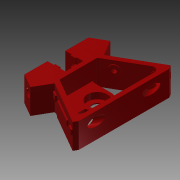
# Autodesk Inventor part: top corner
Saved by Autodesk Inventor 2015 SP1 (Build 190203100, 203)
## iProperties
Created: 2015-01-28
Part Number: top corner
Material: Generic
Document SubType Name: Modeling
Designer: Joseph
Density: 1 g/cm^3
Appearance: Red
Author: Joseph
Autodesk Inventor part; units mm, degrees
note: some values were not read from the file. Chosen so that the rebuilt part matches the saved one: direction of "Hole8".
sketch "Sketch1" plane through (0, 0, 0) normal (0, 0, 1) x (1, 0, 0)
  line L0 (7.9588, 40.9294) -> (17.9588, 23.6089)
  line L1 (17.9588, 23.6089) -> (65.5902, 51.1089)
  line L2 (7.9588, -48.8207) -> (17.9588, -31.5002)
  line L3 (17.9588, -31.5002) -> (65.5902, -59.0002)
  line L4 (65.5902, -59.0002) -> (68.0902, -54.6701)
  line L5 (65.5902, 51.1089) -> (68.0902, 46.7788)
  line L6 (17.039, 17.3044) -> (17.039, -25.1956)
  line L7 (-7.6578, 31.9131) -> (7.9588, 40.9294)
  line L8 (7.9588, -48.8207) -> (-7.6578, -39.8044)
  line L9 (63.0902, 43.892) -> (63.0902, -51.7833)
  line L10 (68.0902, 46.7788) -> (68.0902, -54.6701)
  line L11 (63.0902, 43.892) -> (17.039, 17.3044)
  line L12 (63.0902, -51.7833) -> (17.039, -25.1956)
  line L13 (63.0902, -12.2336) -> (68.0902, -12.2336) construction
  line L14 (63.0902, -51.7833) -> (60.5902, -56.1134) construction
  line L15 (63.0902, 43.892) -> (60.5902, 48.2222) construction
  line L16 (17.039, -3.9456) -> (63.0902, -3.9456) construction
  line L17 (-7.6578, 6.0639) -> (-7.6578, -13.9552) construction
  line L18 (-7.6578, 31.9131) -> (-7.6578, 6.0639)
  line L19 (-7.6578, -13.9552) -> (-7.6578, -39.8044)
  line L20 (-7.6578, -13.9552) -> (-0.4078, -13.9552)
  line L21 (5.0922, -13.9361) -> (12.3422, -13.9361)
  line L22 (12.3422, 6.0639) -> (5.0922, 6.0639)
  line L23 (-0.4078, 6.0639) -> (-7.6578, 6.0639)
  line L24 (12.3422, -6.6861) -> (10.8613, -6.6861)
  line L25 (10.8613, -6.6861) -> (10.8613, -1.1861)
  line L26 (10.8613, -1.1861) -> (12.3422, -1.1861)
  line L27 (5.0922, 6.0639) -> (5.0922, 4.5831)
  line L28 (5.0922, 4.5831) -> (-0.4078, 4.5831)
  line L29 (-0.4078, 4.5831) -> (-0.4078, 6.0639)
  line L30 (-0.4078, -13.9552) -> (-0.4078, -12.4552)
  line L31 (-0.4078, -12.4552) -> (5.0922, -12.4552)
  line L32 (5.0922, -12.4552) -> (5.0922, -13.9361)
  line L33 (12.3422, -13.9361) -> (12.3422, -6.6861)
  line L34 (12.3422, -1.1861) -> (12.3422, 6.0639)
  dimension "d11" = 20
  dimension "d12" = 55
  dimension "d110" = 42.5
  dimension "d176" = 5
  dimension "d177" = 60
  dimension "d178" = 120
  dimension "d179" = 60
  dimension "d181" = 20
  dimension "d184" = 1.5
  dimension "d185" = 5.5
  dimension "d186" = 20
  dimension "d195" = 34.8655
  dimension "d209" = 55
  constraints: 70 end point, 19 perpendicular, 15 equal length, 12 parallel, 6 point on line, 2 horizontal, 2 midpoint
  measures "d11" distance of L2.start L2.end
  measures "d12" distance of L2.end L3.end
  measures "d110" distance of L6.start L6.end
  measures "d176" distance of L3.end L4.end
  measures "d177" angle of L11 L12
  measures "d178" angle of L6 L12
  measures "d179" angle of L1 L3
  measures "d181" distance of L22.start L21.end
  measures "d184" distance of L20.end L30.end
  measures "d185" distance of L30.end L31.end
  measures "d186" distance between parallel lines of L17 L33
  measures "d195" distance from line of L0.start L22
  measures "d209" distance of L0.end L1.end
extrude "Extrusion13" add sketch "Sketch1" along normal blind 20
fillet "Fillet5" radius 5 2 edges at (63.0902, -51.7833, 10) (63.0902, 43.892, 10)
sketch "Sketch2" plane through (7.9588, 40.9294, 20) normal (0.8660254, 0.5, 0) x (0, 0, -1)
  line L0 (20, -20) -> (0, -20) construction
  circle A0 centre (10, -10) radius 10 construction
  circle A1 centre (10, -10) radius 10 construction
  line L1 (7, -21) -> (13, -21)
  line L2 (13, -21) -> (13, -19)
  line L3 (13, -19) -> (7, -19)
  line L4 (7, -19) -> (7, -21)
  line L5 (7, -21) -> (13, -19) construction
  line L6 (13, -21) -> (7, -19) construction
  line L7 (12.8625, -20.9991) -> (6.8625, -20.9991)
  line L8 (6.8625, -20.9991) -> (6.8625, -18.9991)
  line L9 (6.8625, -18.9991) -> (12.8625, -18.9991)
  line L10 (12.8625, -18.9991) -> (12.8625, -20.9991)
  line L11 (12.8625, -20.9991) -> (6.8625, -18.9991) construction
  line L12 (6.8625, -20.9991) -> (12.8625, -18.9991) construction
  line L13 (20, 0) -> (20, -20) projected
  line L14 (0, -20) -> (0, 0) projected
  line L15 (20, -20) -> (0, -20) projected
  point P0 (60, -34.2995)
  point P1 (10, -20)
  point P2 (9.8625, -19.9991)
  dimension "d168" = 20
  dimension "d179" = 60
  dimension "d186" = 20
  dimension "d195" = 34.8655
  dimension "d209" = 55
  dimension "d19" = 20
  dimension "d23" = 6
  dimension "d24" = 2
  dimension "d25" = 6
  dimension "d26" = 2
  constraints: 26 end point, 5 horizontal, 4 midpoint, 4 parallel, 2 perpendicular, 2 vertical, 1 vertical alignment, 5 other
  measures "d19" distance of L0.start L0.end
  measures "d23" distance of L3.end L2.end
  measures "d24" distance of L2.end L1.end
  measures "d25" distance of L8.end L9.end
  measures "d26" distance of L7.end L8.end
extrude "Extrusion2" add sketch "Sketch2" along normal up to surface (55 mm away) from surface at 0
sketch "Sketch8" plane through (17.9588, -31.5002, 20) normal (0.8660254, -0.5, 0) x (0, 0, -1)
  line L0 (0, 0) -> (20, 0) construction
  line L1 (20, 0) -> (0, 0) construction
  line L2 (60, 0) -> (0, 0)
  line L3 (20, 0) -> (0, 0) construction
  line L4 (40, 0) -> (60, 0) construction
  line L5 (20, 0) -> (20, -20) projected
  circle A0 centre (10, -10) radius 10 construction
  line L6 (20, 0) -> (0, 0) projected
  line L7 (10, 0) -> (10, -20) construction
  line L8 (20, -20) -> (0, -20) construction
  line L9 (10, -20) -> (10, 0) construction
  line L10 (12.75, 1.5) -> (7.25, 1.5)
  line L11 (7.25, 1.5) -> (7.25, -1.5)
  line L12 (7.25, -1.5) -> (12.75, -1.5)
  line L13 (12.75, -1.5) -> (12.75, 1.5)
  line L14 (12.75, 1.5) -> (7.25, -1.5) construction
  line L15 (7.25, 1.5) -> (12.75, -1.5) construction
  line L16 (10, 0) -> (10, -20) construction
  line L17 (7.25, -1.5) -> (12.75, -1.5)
  line L18 (12.75, -1.5) -> (12.75, 1.5)
  line L19 (12.75, 1.5) -> (7.25, 1.5)
  line L20 (7.25, 1.5) -> (7.25, -1.5)
  line L21 (7.25, -1.5) -> (12.75, 1.5) construction
  line L22 (12.75, -1.5) -> (7.25, 1.5) construction
  point P0 (60, 16.0535)
  point P1 (60, 3.2816)
  dimension "d169" = 20
  dimension "d171" = 5.5
  dimension "d172" = 3
  dimension "d173" = 5.5
  dimension "d174" = 3
  constraints: 40 end point, 7 midpoint, 4 horizontal, 4 parallel, 2 perpendicular, 2 point on circle, 2 symmetric about line, 2 tangent, 1 centre point, 1 line through centre, 1 vertical
  measures "d169" diameter of A0
  measures "d171" distance of L12.end L11.end
  measures "d172" distance of L11.end L10.end
  measures "d173" distance of L19.end L18.end
  measures "d174" distance of L18.end L17.end
extrude "Extrusion7" add sketch "Sketch8" along normal up to surface (55 mm away) from surface at 0
ref_plane "Work Plane20" through (33.539, 3.3832, 20) normal (0.5, 0.8660254, 0) x (0.8660254, -0.5, 0)
sketch "Sketch9" plane through (33.539, 3.3832, 20) normal (0.5, 0.8660254, 0) x (0.8660254, -0.5, 0)
  line L0 (58.9488, 10) -> (1.9893, 10) construction
  line L1 (48.9488, 10) -> (13.9488, 10) construction
  line L2 (13.9488, 10) -> (13.9488, 10) construction
  line L3 (13.9488, 10) -> (48.9488, 10) construction
  line L4 (48.9488, 10) -> (48.9488, 10) construction
  line L5 (58.9488, 12.75) -> (58.9488, 7.25) construction
  line L6 (58.9488, 12.75) -> (58.9488, 7.25) construction
  line L7 (48.9488, 10) -> (58.9488, 10) construction
  point P0 (-26.8584, -7)
  dimension "d73" = 35
  dimension "d205" = 10
  constraints: 12 end point, 4 coincident, 2 collinear, 2 horizontal, 2 midpoint, 1 parallel, 1 perpendicular, 1 point on line
  measures "d73" distance of L1.end L7.start
  measures "d205" distance of L7.start L7.end
hole "Hole2" at (75.93, -21.0912, 10) at (45.6191, -3.5912, 10) direction (-0.5, -0.8660254, 0) diameter 4.5 end through all counterbore diameter 10 counterbore depth 32.5 clearance for "Socket Head Cap Screw" size "M4" standard "Ansi Metric M Profile"
ref_plane "Work Plane21" through (33.539, -11.2745, 0) normal (0.5, -0.8660254, 0) x (0.8660254, 0.5, 0)
sketch "Sketch10" plane through (33.539, -11.2745, 0) normal (0.5, -0.8660254, 0) x (0.8660254, 0.5, 0)
  line L0 (13.9488, 7.0687) -> (13.9488, 10.1375) construction
  line L1 (13.9488, 10.1375) -> (48.9488, 10.1375) construction
  line L2 (48.9488, 10.1375) -> (48.9488, 7.0687) construction
  line L3 (58.9488, 13.1375) -> (58.9488, 7.1375) construction
  line L4 (58.6448, 7.1375) -> (58.6448, 7) construction
  line L5 (48.9488, 10.1375) -> (58.9488, 10.1375) construction
  point P0 (-25.1395, 13)
  point P1 (60.4691, 53)
  point P2 (58.6448, 7.1375)
  dimension "d74" = 35
  dimension "d208" = 10
  constraints: 8 end point, 2 coincident, 1 collinear, 1 midpoint, 1 parallel, 3 other
  measures "d74" distance of L1.end L0.end
  measures "d208" distance between parallel lines of L2 L3
hole "Hole3" at (75.93, 13.1999, 10.1375) at (45.6191, -4.3001, 10.1375) direction (-0.5, 0.8660254, 0) diameter 4.5 end through all counterbore diameter 10 counterbore depth 32.5 clearance for "Socket Head Cap Screw" size "M4" standard "Ansi Metric M Profile"
ref_plane "Work Plane18" through (7.9588, 40.9294, 0) normal (0, -1, 0) x (1, 0, 0)
sketch "Sketch20" plane through (7.9588, 40.9294, 0) normal (0, -1, 0) x (1, 0, 0)
  line L0 (-2.8667, 0) -> (-8.3667, 0) construction
  line L1 (-8.3667, 20) -> (-2.8667, 20) construction
  line L2 (-5.6167, 0) -> (-5.6167, 20) construction
  point P0 (-7.9588, 0)
  point P1 (-5.6167, 10)
  constraints: 3 midpoint, 2 end point
hole "Hole7" at (2.3422, 40.9294, 10) direction (0, -1, 0) diameter 4.5 end up to surface counterbore diameter 8 counterbore depth 16.35 clearance for "Socket Head Cap Screw" size "M4" standard "Ansi Metric M Profile"
ref_plane "Work Plane19" through (7.9588, -48.8207, 0) normal (0, -1, 0) x (1, 0, 0)
sketch "Sketch21" plane through (7.9588, -48.8207, 0) normal (0, -1, 0) x (1, 0, 0)
  line L0 (-8.3667, 0) -> (-2.8667, 0) projected
  line L1 (-2.8667, 20) -> (-8.3667, 20) projected
  line L2 (-5.6167, 20) -> (-5.6167, 0) construction
  point P0 (-7.9588, 0)
  point P1 (-5.6167, 10)
  constraints: 3 midpoint, 2 end point
hole "Hole8" at (2.3422, -48.8207, 10) direction (0, 1, 0) diameter 4.5 end up to surface counterbore diameter 8 counterbore depth 16.35 clearance for "Socket Head Cap Screw" size "M4" standard "Ansi Metric M Profile"
fillet "Fillet6" radius 2 4 edges at (17.039, 17.3044, 10) (17.039, -25.1956, 10) (68.0902, -54.6701, 10) (68.0902, 46.7788, 10)
sketch "Sketch22" plane through (55.5902, -47.4532, 20) normal (0.5, 0.8660254, 0) x (0.8660254, -0.5, 0)
  circle A0 centre (-30.5662, 10) radius 2.25 projected
  circle A1 centre (4.4338, 10) radius 2.25 projected
  circle A2 centre (-30.5662, 10) radius 6
  circle A3 centre (4.4338, 10) radius 6
  point P0 (-71.8691, 20)
  dimension "d211" = 12
  dimension "d212" = 12
  constraints: 2 centre point, 2 coincident
  measures "d211" diameter of A2
  measures "d212" diameter of A3
extrude "Extrusion14" add sketch "Sketch22" along normal blind 1
sketch "Sketch23" plane through (55.5902, 39.5619, 0) normal (0.5, -0.8660254, 0) x (0.8660254, 0.5, 0)
  circle A0 centre (-30.5662, 10.1375) radius 2.25 projected
  circle A1 centre (4.4338, 10.1375) radius 2.25 projected
  circle A2 centre (-30.5662, 10.1375) radius 6
  circle A3 centre (4.4338, 10.1375) radius 6
  point P0 (-67.9235, 0)
  dimension "d215" = 12
  dimension "d216" = 12
  constraints: 2 centre point, 2 coincident
  measures "d215" diameter of A2
  measures "d216" diameter of A3
extrude "Extrusion15" add sketch "Sketch23" along normal blind 1
sketch "Sketch24" plane through (17.2088, -32.7992, 7.25) normal (-0.5, -0.8660254, 0) x (0.8660254, -0.5, 0)
  circle A0 centre (45, 2.75) radius 2.25 projected
  circle A1 centre (10, 2.75) radius 2.25 projected
  line L0 (6.875, 5.875) -> (13.125, 5.875)
  line L1 (13.125, 5.875) -> (13.125, -0.375)
  line L2 (13.125, -0.375) -> (6.875, -0.375)
  line L3 (6.875, -0.375) -> (6.875, 5.875)
  line L4 (6.875, 5.875) -> (13.125, -0.375) construction
  line L5 (13.125, 5.875) -> (6.875, -0.375) construction
  line L6 (41.875, 5.875) -> (48.125, 5.875)
  line L7 (48.125, 5.875) -> (48.125, -0.375)
  line L8 (48.125, -0.375) -> (41.875, -0.375)
  line L9 (41.875, -0.375) -> (41.875, 5.875)
  line L10 (41.875, 5.875) -> (48.125, -0.375) construction
  line L11 (48.125, 5.875) -> (41.875, -0.375) construction
  point P0 (-31.3029, -7.25)
  dimension "d219" = 6.25
  dimension "d220" = 6.25
  dimension "d221" = 6.25
  dimension "d222" = 6.25
  constraints: 24 end point, 4 midpoint, 4 parallel, 2 horizontal, 2 perpendicular
  measures "d219" distance of L1.end L2.end
  measures "d220" distance of L0.end L1.end
  measures "d221" distance of L7.end L8.end
  measures "d222" distance of L6.end L7.end
extrude "Extrusion16" cut sketch "Sketch24" against normal up to surface (1.5 mm away)
sketch "Sketch25" plane through (17.4584, 24.4757, 13.1375) normal (-0.5, 0.8660254, 0) x (0.8660254, 0.5, 0)
  circle A0 centre (45, 3) radius 2.25 projected
  circle A1 centre (10, 3) radius 2.25 projected
  line L0 (6.875, -0.125) -> (13.125, -0.125)
  line L1 (13.125, -0.125) -> (13.125, 6.125)
  line L2 (13.125, 6.125) -> (6.875, 6.125)
  line L3 (6.875, 6.125) -> (6.875, -0.125)
  line L4 (6.875, -0.125) -> (13.125, 6.125) construction
  line L5 (13.125, -0.125) -> (6.875, 6.125) construction
  line L6 (41.875, -0.125) -> (48.125, -0.125)
  line L7 (48.125, -0.125) -> (48.125, 6.125)
  line L8 (48.125, 6.125) -> (41.875, 6.125)
  line L9 (41.875, 6.125) -> (41.875, -0.125)
  line L10 (41.875, -0.125) -> (48.125, 6.125) construction
  line L11 (48.125, -0.125) -> (41.875, 6.125) construction
  point P0 (-27.3573, 13.1375)
  dimension "d225" = 6.25
  dimension "d226" = 6.25
  dimension "d227" = 6.25
  dimension "d228" = 6.25
  constraints: 24 end point, 4 midpoint, 4 parallel, 2 horizontal, 2 perpendicular
  measures "d225" distance of L2.end L1.end
  measures "d226" distance of L1.end L0.end
  measures "d227" distance of L8.end L7.end
  measures "d228" distance of L7.end L6.end
extrude "Extrusion17" cut sketch "Sketch25" against normal up to surface (1.0009 mm away)
sketch "Sketch26" plane through (-0.4078, -12.4552, 0) normal (0, 1, 0) x (1, 0, 0)
  circle A0 centre (2.75, -10) radius 2.25 projected
  line L0 (5.875, -13.125) -> (-0.375, -13.125)
  line L1 (-0.375, -13.125) -> (-0.375, -6.875)
  line L2 (-0.375, -6.875) -> (5.875, -6.875)
  line L3 (5.875, -6.875) -> (5.875, -13.125)
  line L4 (5.875, -13.125) -> (-0.375, -6.875) construction
  line L5 (-0.375, -13.125) -> (5.875, -6.875) construction
  point P0 (0.4078, 0)
  dimension "d231" = 6.25
  dimension "d232" = 6.25
  constraints: 12 end point, 2 midpoint, 2 parallel, 1 horizontal, 1 perpendicular
  measures "d231" distance of L1.end L2.end
  measures "d232" distance of L0.end L1.end
extrude "Extrusion18" cut sketch "Sketch26" against normal up to surface (1.5 mm away)
sketch "Sketch27" plane through (-0.4078, 4.5831, 0) normal (0, -1, 0) x (1, 0, 0)
  circle A0 centre (2.75, 10) radius 2.25 projected
  line L0 (5.875, 13.125) -> (-0.375, 13.125)
  line L1 (-0.375, 13.125) -> (-0.375, 6.875)
  line L2 (-0.375, 6.875) -> (5.875, 6.875)
  line L3 (5.875, 6.875) -> (5.875, 13.125)
  line L4 (5.875, 13.125) -> (-0.375, 6.875) construction
  line L5 (-0.375, 13.125) -> (5.875, 6.875) construction
  point P0 (0.4078, 0)
  dimension "d235" = 6.25
  dimension "d236" = 6.25
  constraints: 12 end point, 2 midpoint, 2 parallel, 1 horizontal, 1 perpendicular
  measures "d235" distance of L2.end L1.end
  measures "d236" distance of L1.end L0.end
extrude "Extrusion19" cut sketch "Sketch27" against normal up to surface (1.4809 mm away)
sketch "Sketch28" plane through (0, 0, 0) normal (0, 0, -1) x (-1, 0, 0)
  line L0 (-55.5902, 39.5619) -> (-18.039, 17.8817) projected
  arc A0 (-17.039, 16.1497) -> (-18.039, 17.8817) centre (-19.039, 16.1497) ccw projected
  line L1 (-17.039, 16.1497) -> (-17.039, -24.0409) projected
  arc A1 (-18.039, -25.773) -> (-17.039, -24.0409) centre (-19.039, -24.0409) ccw projected
  line L2 (-18.039, -25.773) -> (-55.5902, -47.4532) projected
  arc A2 (-63.0902, -43.1231) -> (-55.5902, -47.4532) centre (-58.0902, -43.1231) ccw projected
  line L3 (-63.0902, -43.1231) -> (-63.0902, 35.2318) projected
  arc A3 (-55.5902, 39.5619) -> (-63.0902, 35.2318) centre (-58.0902, 35.2318) ccw projected
  arc A4 (-67.8223, 47.2429) -> (-68.0902, 46.2429) centre (-66.0902, 46.2429) ccw projected
  line L4 (-68.0902, 46.2429) -> (-68.0902, -54.1342) projected
  arc A5 (-68.0902, -54.1342) -> (-67.8223, -55.1342) centre (-66.0902, -54.1342) ccw projected
  line L5 (-67.8223, -55.1342) -> (-65.5902, -59.0002) projected
  line L6 (-65.5902, -59.0002) -> (-17.9588, -31.5002) projected
  line L7 (-17.9588, -31.5002) -> (-7.9588, -48.8207) projected
  line L8 (7.6578, -13.9552) -> (0.4078, -13.9552) projected
  line L9 (0.4078, -13.9552) -> (0.4078, -12.4552) projected
  line L10 (-5.0922, -12.4552) -> (-5.0922, -13.9361) projected
  line L11 (-5.0922, -13.9361) -> (-12.3422, -13.9361) projected
  line L12 (-12.3422, -13.9361) -> (-12.3422, -6.6861) projected
  line L13 (-12.3422, -6.6861) -> (-10.8613, -6.6861) projected
  line L14 (-10.8613, -6.6861) -> (-10.8613, -1.1861) projected
  line L15 (-10.8613, -1.1861) -> (-12.3422, -1.1861) projected
  line L16 (-12.3422, -1.1861) -> (-12.3422, 6.0639) projected
  line L17 (-12.3422, 6.0639) -> (-5.0922, 6.0639) projected
  line L18 (-5.0922, 6.0639) -> (-5.0922, 4.5831) projected
  line L19 (-5.0922, 4.5831) -> (0.4078, 4.5831) projected
  line L20 (0.4078, 4.5831) -> (0.4078, 6.0639) projected
  line L21 (0.4078, 6.0639) -> (7.6578, 6.0639) projected
  line L22 (7.6578, 6.0639) -> (7.6578, 31.9131) projected
  line L23 (7.6578, 31.9131) -> (-7.9588, 40.9294) projected
  line L24 (-7.9588, 40.9294) -> (-17.9588, 23.6089) projected
  line L25 (-17.9588, 23.6089) -> (-65.5902, 51.1089) projected
  line L26 (-65.5902, 51.1089) -> (-67.8223, 47.2429) projected
  circle A6 centre (-38.289, -3.945) radius 4 projected
  line L27 (-7.9588, -48.8207) -> (7.6578, -39.8044) projected
  line L28 (7.6578, -39.8044) -> (7.6578, -13.9552) projected
  line L29 (7.1578, -13.9552) -> (0.2857, -13.9552) projected
  line L30 (0.4078, -12.4552) -> (-5.0922, -12.4552) projected
  circle A7 centre (-38.289, -3.945) radius 11.25
  line L31 (-38.289, 11.055) -> (-17.039, 11.055)
  line L32 (-17.039, -18.945) -> (-38.289, -18.945)
  line L33 (-63.0902, -7.945) -> (-52.7459, -7.945)
  line L34 (-63.0902, 0.055) -> (-52.7459, 0.055)
  arc A8 (-38.289, 11.055) -> (-52.7459, 0.055) centre (-38.289, -3.945) ccw
  arc A9 (-52.7459, -7.945) -> (-38.289, -18.945) centre (-38.289, -3.945) ccw
  point P0 (0, 0)
  dimension "d239" = 22.5
  constraints: 8 end point, 4 point on circle, 4 point on line, 3 centre point, 3 perpendicular, 2 coincident, 2 parallel, 1 tangent, 1 other
  measures "d239" diameter of A7
extrude "Extrusion20" add sketch "Sketch28" along normal blind 7 contours L34 A8 L31 L1 L32 A9 L33 L3 | L26 L25 L24 L23 L22 L21 L20 L19 L18 L17 L16 L15 L14 L13 L12 L11 L10 L30 L9 L8 L28 L27 L7 L6 L5 A5 L4 A4
sketch "Sketch29" plane through (0, 0, -7) normal (0, 0, -1) x (-1, 0, 0)
  arc A0 (-18.039, -25.773) -> (-17.039, -24.0409) centre (-19.039, -24.0409) ccw projected
  line L0 (-18.039, -25.773) -> (-55.5902, -47.4532) projected
  arc A1 (-63.0902, -43.1231) -> (-55.5902, -47.4532) centre (-58.0902, -43.1231) ccw projected
  line L1 (-63.0902, -43.1231) -> (-63.0902, -7.945) projected
  line L2 (-63.0902, -7.945) -> (-52.7459, -7.945) projected
  arc A2 (-52.7459, -7.945) -> (-38.289, -18.945) centre (-38.289, -3.945) ccw projected
  line L3 (-38.289, -18.945) -> (-17.039, -18.945) projected
  line L4 (-17.039, -18.945) -> (-17.039, -24.0409) projected
  line L5 (-55.5902, 39.5619) -> (-18.039, 17.8817) projected
  arc A3 (-17.039, 16.1497) -> (-18.039, 17.8817) centre (-19.039, 16.1497) ccw projected
  line L6 (-17.039, 16.1497) -> (-17.039, 11.055) projected
  line L7 (-17.039, 11.055) -> (-38.289, 11.055) projected
  arc A4 (-38.289, 11.055) -> (-52.7459, 0.055) centre (-38.289, -3.945) ccw projected
  line L8 (-52.7459, 0.055) -> (-63.0902, 0.055) projected
  line L9 (-63.0902, 0.055) -> (-63.0902, 35.2318) projected
  arc A5 (-55.5902, 39.5619) -> (-63.0902, 35.2318) centre (-58.0902, 35.2318) ccw projected
  arc A6 (-67.8223, 47.2429) -> (-68.0902, 46.2429) centre (-66.0902, 46.2429) ccw projected
  line L10 (-68.0902, 46.2429) -> (-68.0902, -54.1342) projected
  arc A7 (-68.0902, -54.1342) -> (-67.8223, -55.1342) centre (-66.0902, -54.1342) ccw projected
  line L11 (-67.8223, -55.1342) -> (-65.5902, -59.0002) projected
  line L12 (-65.5902, -59.0002) -> (-17.9588, -31.5002) projected
  line L13 (-17.9588, -31.5002) -> (-7.9588, -48.8207) projected
  line L14 (-7.9588, -48.8207) -> (7.6578, -39.8044) projected
  line L15 (7.6578, -39.8044) -> (7.6578, -13.9552) projected
  line L16 (7.6578, -13.9552) -> (0.4078, -13.9552) projected
  line L17 (0.4078, -13.9552) -> (0.4078, -12.4552) projected
  line L18 (0.4078, -12.4552) -> (-5.0922, -12.4552) projected
  line L19 (-5.0922, -12.4552) -> (-5.0922, -13.9361) projected
  line L20 (-5.0922, -13.9361) -> (-12.3422, -13.9361) projected
  line L21 (-12.3422, -13.9361) -> (-12.3422, -6.6861) projected
  line L22 (-12.3422, -6.6861) -> (-10.8613, -6.6861) projected
  line L23 (-10.8613, -6.6861) -> (-10.8613, -1.1861) projected
  line L24 (-10.8613, -1.1861) -> (-12.3422, -1.1861) projected
  line L25 (-12.3422, -1.1861) -> (-12.3422, 6.0639) projected
  line L26 (-12.3422, 6.0639) -> (-5.0922, 6.0639) projected
  line L27 (-5.0922, 6.0639) -> (-5.0922, 4.5831) projected
  line L28 (-5.0922, 4.5831) -> (0.4078, 4.5831) projected
  line L29 (0.4078, 4.5831) -> (0.4078, 6.0639) projected
  line L30 (0.4078, 6.0639) -> (7.6578, 6.0639) projected
  line L31 (7.6578, 6.0639) -> (7.6578, 31.9131) projected
  line L32 (7.6578, 31.9131) -> (-7.9588, 40.9294) projected
  line L33 (-7.9588, 40.9294) -> (-17.9588, 23.6089) projected
  line L34 (-17.9588, 23.6089) -> (-65.5902, 51.1089) projected
  line L35 (-65.5902, 51.1089) -> (-67.8223, 47.2429) projected
  circle A8 centre (-38.289, -3.945) radius 6
  point P0 (0, 0)
  dimension "d243" = 12
  constraints: 1 centre point, 1 coincident
  measures "d243" diameter of A8
extrude "Extrusion21" add sketch "Sketch29" along normal blind 1
fillet "Fillet7" radius 2 6 edges at (52.7459, -7.945, -4) (17.039, -18.945, -4) (52.7459, 0.055, -4) (17.039, 11.055, -4) (63.0902, -7.945, -4) (63.0902, 0.055, -4)
sketch "Sketch30" plane through (0, 0, -8) normal (0, 0, -1) x (-1, 0, 0)
  line L0 (-18.039, -25.773) -> (-55.5902, -47.4532) projected
  arc A0 (-52.3237, -9.2391) -> (-38.289, -18.945) centre (-38.289, -3.945) ccw projected
  line L1 (-38.289, -18.945) -> (-19.039, -18.945) projected
  arc A1 (-17.039, -20.945) -> (-19.039, -18.945) centre (-19.039, -20.945) ccw projected
  line L2 (-17.039, -20.945) -> (-17.039, -24.0409) projected
  arc A2 (-18.039, -25.773) -> (-17.039, -24.0409) centre (-19.039, -24.0409) ccw projected
  line L3 (-39.6795, -38.2671) -> (-39.6795, -18.8804)
  point P0 (0, 0)
  constraints: 2 end point, 1 point on circle, 1 point on line, 1 vertical
extrude "Extrusion22" add sketch "Sketch30" against normal up to surface (8 mm away)
fillet "Fillet8" radius 2 2 edges at (39.6795, -18.8804, -4) (39.6795, -38.2671, -4)
sketch "Sketch31" plane through (0, 0, -8) normal (0, 0, -1) x (-1, 0, 0)
  circle A0 centre (-35.6338, -29.963) radius 1.535
  circle A1 centre (-16.7038, -29.963) radius 1.535
  point P0 (0, 0)
  constraints: 2 centre point, 2 coincident, 4 other
hole "Hole9" at (35.6338, -29.963, -8) at (16.7038, -29.963, -8) direction (0, 0, 1) diameter 3 depth 12 tip angle 118
sketch "Sketch32" plane through (0, 0, -8) normal (0, 0, -1) x (-1, 0, 0)
  circle A0 centre (-35.6338, -29.963) radius 1.5 projected
  circle A1 centre (-16.7038, -29.963) radius 1.5 projected
  circle A2 centre (-35.6338, -29.963) radius 1.5 projected
  circle A3 centre (-16.7038, -29.963) radius 1.5 projected
  circle A4 centre (-38.289, -3.945) radius 6 projected
  line L0 (-40.6795, -38.8445) -> (-55.5902, -47.4532) projected
  arc A5 (-63.0902, -43.1231) -> (-55.5902, -47.4532) centre (-58.0902, -43.1231) ccw projected
  line L1 (-63.0902, -43.1231) -> (-63.0902, -9.945) projected
  arc A6 (-61.0902, -7.945) -> (-63.0902, -9.945) centre (-61.0902, -9.945) ccw projected
  line L2 (-61.0902, -7.945) -> (-54.195, -7.945) projected
  arc A7 (-52.3237, -9.2391) -> (-54.195, -7.945) centre (-54.195, -9.945) ccw projected
  arc A8 (-52.3237, -9.2391) -> (-41.2806, -18.6436) centre (-38.289, -3.945) ccw projected
  arc A9 (-39.6795, -20.6034) -> (-41.2806, -18.6436) centre (-41.6795, -20.6034) ccw projected
  line L3 (-39.6795, -20.6034) -> (-39.6795, -37.1124) projected
  arc A10 (-40.6795, -38.8445) -> (-39.6795, -37.1124) centre (-41.6795, -37.1124) ccw projected
  arc A11 (-17.039, 16.1497) -> (-18.039, 17.8817) centre (-19.039, 16.1497) ccw projected
  line L4 (-17.039, 16.1497) -> (-17.039, 13.055) projected
  arc A12 (-19.039, 11.055) -> (-17.039, 13.055) centre (-19.039, 13.055) ccw projected
  line L5 (-19.039, 11.055) -> (-38.289, 11.055) projected
  arc A13 (-38.289, 11.055) -> (-52.3237, 1.3492) centre (-38.289, -3.945) ccw projected
  arc A14 (-54.195, 0.055) -> (-52.3237, 1.3492) centre (-54.195, 2.055) ccw projected
  line L6 (-54.195, 0.055) -> (-61.0902, 0.055) projected
  arc A15 (-63.0902, 2.055) -> (-61.0902, 0.055) centre (-61.0902, 2.055) ccw projected
  line L7 (-63.0902, 2.055) -> (-63.0902, 35.2318) projected
  arc A16 (-55.5902, 39.5619) -> (-63.0902, 35.2318) centre (-58.0902, 35.2318) ccw projected
  line L8 (-55.5902, 39.5619) -> (-18.039, 17.8817) projected
  arc A17 (-67.8223, 47.2429) -> (-68.0902, 46.2429) centre (-66.0902, 46.2429) ccw projected
  line L9 (-68.0902, 46.2429) -> (-68.0902, -54.1342) projected
  arc A18 (-68.0902, -54.1342) -> (-67.8223, -55.1342) centre (-66.0902, -54.1342) ccw projected
  line L10 (-67.8223, -55.1342) -> (-65.5902, -59.0002) projected
  line L11 (-65.5902, -59.0002) -> (-17.9588, -31.5002) projected
  line L12 (-17.9588, -31.5002) -> (-7.9588, -48.8207) projected
  line L13 (-7.9588, -48.8207) -> (7.6578, -39.8044) projected
  line L14 (7.6578, -39.8044) -> (7.6578, -13.9552) projected
  line L15 (7.6578, -13.9552) -> (0.4078, -13.9552) projected
  line L16 (0.4078, -13.9552) -> (0.4078, -12.4552) projected
  line L17 (0.4078, -12.4552) -> (-5.0922, -12.4552) projected
  line L18 (-5.0922, -12.4552) -> (-5.0922, -13.9361) projected
  line L19 (-5.0922, -13.9361) -> (-12.3422, -13.9361) projected
  line L20 (-12.3422, -13.9361) -> (-12.3422, -6.6861) projected
  line L21 (-12.3422, -6.6861) -> (-10.8613, -6.6861) projected
  line L22 (-10.8613, -6.6861) -> (-10.8613, -1.1861) projected
  line L23 (-10.8613, -1.1861) -> (-12.3422, -1.1861) projected
  line L24 (-12.3422, -1.1861) -> (-12.3422, 6.0639) projected
  line L25 (-12.3422, 6.0639) -> (-5.0922, 6.0639) projected
  line L26 (-5.0922, 6.0639) -> (-5.0922, 4.5831) projected
  line L27 (-5.0922, 4.5831) -> (0.4078, 4.5831) projected
  line L28 (0.4078, 4.5831) -> (0.4078, 6.0639) projected
  line L29 (0.4078, 6.0639) -> (7.6578, 6.0639) projected
  line L30 (7.6578, 6.0639) -> (7.6578, 31.9131) projected
  line L31 (7.6578, 31.9131) -> (-7.9588, 40.9294) projected
  line L32 (-7.9588, 40.9294) -> (-17.9588, 23.6089) projected
  line L33 (-17.9588, 23.6089) -> (-65.5902, 51.1089) projected
  line L34 (-65.5902, 51.1089) -> (-67.8223, 47.2429) projected
  line L35 (-46.7588, -25.043) -> (-13.8688, -25.043)
  line L36 (-13.8688, -35.043) -> (-46.7588, -35.043)
  line L37 (-33.1338, -25.043) -> (-19.2038, -25.043)
  line L38 (-19.2038, -25.043) -> (-19.2038, -35.043)
  line L39 (-19.2038, -35.043) -> (-33.1338, -35.043)
  line L40 (-33.1338, -35.043) -> (-33.1338, -25.043)
  point P0 (0, 0)
  dimension "d257" = 1
  dimension "d258" = 1
  constraints: 12 end point, 3 horizontal, 2 parallel, 2 point on line, 1 perpendicular, 4 other
  measures "d257" distance edge to line of A0 L40
  measures "d258" distance edge to line of A1 L38
extrude "Extrusion23" cut sketch "Sketch32" against normal blind 1.5 contours L40 L35 L38 L11 L36 | L11 L38 L36
body "Solid1"
body "Solid2"
